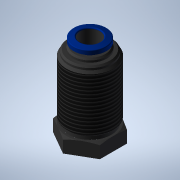
# Autodesk Inventor part: 189199 ESH-HA-4-QS
Saved by Autodesk Inventor 2021 (Build 250183000, 183)
## iProperties
Created: 2026-04-19
Part Number: 189199 ESH-HA-4-QS
Material: Generic
Catalog Web Link: www.3dfindit.com
Description: ESH-HA-...-Suction cup holder
Vendor: FESTO
Document SubType Name: Modeling
Designer: psAdmin
Manufacturer: FESTO
Mass: 3.23763 g
Surface Area: 19.736 cm^2
Volume: 3.23763 cm^3
Density: 1 g/cm^3
Appearance: PSOLRGB-176-176-176
Category: PARTsolutions
Company: FESTO
Title: 189199 ESH-HA-4-QS
Author: Cadenas PARTsolutions
Comments: Suction cup holder
PSOL_IDENT_0: {$CADENAS_DATA/23d-libs/festo/parts/e/esh/parts/esh_ha.prj},180 {VTYP=3D},{NB=189199 ESH-HA-4-QS},{L
PSOL_IDENT_1: INA=189199 ESH-HA-4-QS},{NN=ESH-HA-...},{DATE=17.04.2026 14:02:00},{GEOMDATE=22.08.2023 09:24:42},{V
PSOL_IDENT_2: ERSION=},{LINEID=80},{WBVAR=},{WBNUMERIC=}  {NB=189199 ESH-HA-4-QS},{LINA=189199 ESH-HA-4-QS},{KT=8}
PSOL_IDENT_3: ,{TNR=189199},{TYP=ESH-HA-4-QS},{GR=4},{ZZ=0.1},{ANSCHL=QS},{GEO=8.000},{MN=14.000}
NB: 189199 ESH-HA-4-QS
NN: ESH-HA-...
NT: Suction cup holder
NBSYN: $TNR. $TYP.
LINA: 189199 ESH-HA-4-QS
CATALOG: Festo
TNR: 189199
TYP: ESH-HA-4-QS
ANSCHL: QS
MN: 14
SUPPLIER: FESTO
ARTICLENO: 189199 ESH-HA-4-QS
BOMINFO: 189199 ESH-HA-4-QS
CREATOR: CADENAS GmbH
Autodesk Inventor part; units mm, degrees
sketch "Sketch_2" plane through (0, 0, 0) normal (0, 0, 1) x (1, 0, 0)
  line L0 (0, 0) -> (0, 28)
  line L1 (0, 28) -> (3.3, 28)
  line L2 (3.3, 28) -> (4.7347, 27.747)
  arc A0 (4.9, 27.5501) -> (4.7347, 27.747) centre (4.7, 27.5501) ccw
  line L3 (4.9, 27.5501) -> (4.9, 26.5)
  line L4 (4.9, 26.5) -> (4, 26.5)
  arc A1 (4, 26.5) -> (3.7, 26.2) centre (4, 26.2) ccw
  line L5 (3.7, 26.2) -> (3.7, 25.6)
  line L6 (3.7, 25.6) -> (4.5757, 25.6)
  line L7 (4.5757, 25.6) -> (5, 25.1757)
  line L8 (5, 25.1757) -> (5, 24.6)
  line L9 (5, 24.6) -> (5.9622, 24.6)
  line L10 (5.9622, 24.6) -> (6.3865, 24.1757)
  line L11 (6.3865, 24.1757) -> (6.3865, 23.6)
  line L12 (6.3865, 23.6) -> (7, 22.9865)
  line L13 (7, 22.9865) -> (7, 7.2135)
  line L14 (7, 7.2135) -> (6.3865, 6.6)
  line L15 (6.3865, 6.6) -> (6.3865, 5.6)
  line L16 (6.3865, 5.6) -> (7, 5.6)
  line L17 (7, 5.6) -> (8.4, 5.0904)
  line L18 (8.4, 5.0904) -> (8.4, 1.6)
  line L19 (8.4, 1.6) -> (4.2, 1.6)
  line L20 (4.2, 1.6) -> (4.2, 0)
  line L21 (4.2, 0) -> (0, 0)
  line L22 (0, 0) -> (0, 28)
  constraints: 46 end point, 4 point on circle, 2 centre point
revolve "Revolution1" add sketch "Sketch_2" angle 360 about axis through (0, 0, 0) along (0, -1, 0)
thread "Thread1" size "M14x1" class "6g" standard "ISO Metric profile" full length
sketch "Sketch_3" plane through (0, 0, 0) normal (0, 0, 1) x (1, 0, 0)
  line L0 (0, 0) -> (0, 28)
  line L1 (0, 28) -> (3.3, 28)
  arc A0 (3.3, 28) -> (3, 27.7) centre (3.3, 27.7) ccw
  line L2 (3, 27.7) -> (3, 16)
  line L3 (3, 16) -> (1.5, 16)
  line L4 (1.5, 16) -> (1.5, 12.9585)
  line L5 (1.5, 12.9585) -> (2.4585, 12)
  line L6 (2.4585, 12) -> (2.4585, 0.5415)
  line L7 (2.4585, 0.5415) -> (3, 0)
  line L8 (3, 0) -> (0, 0)
  line L9 (0, 0) -> (0, 28)
  constraints: 20 end point, 2 point on circle, 1 centre point
revolve "Revolution2" cut sketch "Sketch_3" angle 360 about axis through (0, 0, 0) along (0, -1, 0)
thread "Thread2" size "M6x1" class "6H" standard "ISO Metric profile" full length
sketch "Sketch_1" plane through (0, 5.6, 0) normal (0, 1, 0) x (1, 0, 0)
  line L0 (-13.4451, -13.8453) -> (13.2851, -13.8453)
  line L1 (13.2851, -13.8453) -> (13.2851, 13.6852)
  line L2 (13.2851, 13.6852) -> (-13.4451, 13.6852)
  line L3 (-13.4451, 13.6852) -> (-13.4451, -13.8453)
  line L4 (-7, -4.0415) -> (0, -8.0829)
  line L5 (0, -8.0829) -> (7, -4.0415)
  line L6 (7, -4.0415) -> (7, 4.0415)
  line L7 (7, 4.0415) -> (0, 8.0829)
  line L8 (0, 8.0829) -> (-7, 4.0415)
  line L9 (-7, 4.0415) -> (-7, -4.0415)
  constraints: 20 end point
extrude "Extrusion1" cut sketch "Sketch_1" against normal blind 5.6
ref_plane "MUTTER1_XY" through (0, 10, 0) normal (0, 1, 0) x (1, 0, 0)
ref_plane "MUTTER1_YZ" through (0, 10, 0) normal (1, 0, 0) x (0, 0, -1)
ref_plane "MUTTER1_ZX" through (0, 10, 0) normal (0, 0, -1) x (0, 1, 0)
ref_plane "MUTTER2_XY" through (0, 18, 0) normal (0, 1, 0) x (1, 0, 0)
ref_plane "MUTTER2_YZ" through (0, 18, 0) normal (1, 0, 0) x (0, 0, -1)
ref_plane "MUTTER2_ZX" through (0, 18, 0) normal (0, 0, -1) x (0, 1, 0)
ref_plane "Sauger_XY" through (0, 0, 0) normal (0, 1, 0) x (1, 0, 0)
ref_plane "Sauger_YZ" through (0, 0, 0) normal (1, 0, 0) x (0, 0, -1)
ref_plane "Sauger_ZX" through (0, 0, 0) normal (0, 0, -1) x (0, 1, 0)
body "Solid1"
